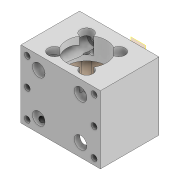
# Autodesk Inventor part: 30_Linear_Captive_Nema8_Guidemount
Saved by Autodesk Inventor 2022 (Build 260153000, 153)
## iProperties
Created: 2022-12-17
Part Number: 30_Linear_Captive_Nema8_Guidemount
Material: Generisch
Document SubType Name: Modeling
Designer: diederichbenedict
Density: 1 g/cm^3
Appearance: Vorgabe
Author: diederichbenedict
Autodesk Inventor part; units mm, degrees
ref_plane "YZ Plane" through (0, 0, 0) normal (1, 0, 0) x (0, 1, 0)
ref_plane "Arbeitsebene1" through (19.299985, 0, -3) normal (0, 0, 1) x (1, 0, 0)
ref_plane "Arbeitsebene2" through (22.999982, -10.5, 0) normal (0, 1, 0) x (-1, 0, 0)
ref_plane "Arbeitsebene3" through (-0.600008, 0, -10) normal (0, 1, 0) x (0, 0, 1)
sketch "Skizze1" plane through (22.999982, -10.5, 0) normal (0, 1, 0) x (-1, 0, 0)
  circle A0 centre (10.1, 12.1) radius 9.4488
  line L0 (0, 19.9) -> (0, 4.3)
  circle A1 centre (2.4, 4.4) radius 1
  circle A2 centre (2.4, 19.8) radius 1
  circle A3 centre (17.8, 19.8) radius 1
  circle A4 centre (17.8, 4.4) radius 1
  arc A5 (4.255177, -11.626563) -> (4.832799, -11.127251) centre (3.800005, -10.516241) ccw
  arc A6 (5.026176, -11.005497) -> (4.832799, -11.127251) centre (5.047965, -11.254545) ccw
  line L1 (5.026176, -11.005497) -> (5.371793, -10.975259)
  arc A7 (5.371793, -10.975259) -> (5.600004, -10.726211) centre (5.350004, -10.726211) ccw
  line L2 (5.600004, -10.726211) -> (5.600004, -10.273789)
  arc A8 (5.600004, -10.273789) -> (5.371793, -10.024741) centre (5.350004, -10.273789) ccw
  line L3 (5.371793, -10.024741) -> (5.005228, -9.992671)
  arc A9 (4.815463, -9.876832) -> (5.005228, -9.992671) centre (5.027016, -9.743622) ccw
  arc A10 (4.815463, -9.876832) -> (4.255177, -9.405918) centre (3.800005, -10.516241) ccw
  arc A11 (4.100005, -9.174601) -> (4.255177, -9.405918) centre (4.350005, -9.174601) ccw
  line L4 (4.100005, -9.174601) -> (4.100005, -8.500004)
  line L5 (4.100005, -8.500004) -> (4.600004, -8.000004)
  line L6 (4.600004, -8.000004) -> (15.599996, -8.000004)
  line L7 (15.599996, -8.000004) -> (16.099995, -8.500004)
  line L8 (16.099995, -8.500004) -> (16.099995, -9.174601)
  arc A12 (15.944823, -9.405918) -> (16.099995, -9.174601) centre (15.849995, -9.174601) ccw
  arc A13 (15.944823, -9.405918) -> (15.384537, -9.876832) centre (16.399995, -10.516241) ccw
  arc A14 (15.194772, -9.992671) -> (15.384537, -9.876832) centre (15.172984, -9.743622) ccw
  line L9 (15.194772, -9.992671) -> (14.828207, -10.024741)
  arc A15 (14.828207, -10.024741) -> (14.599996, -10.273789) centre (14.849996, -10.273789) ccw
  line L10 (14.599996, -10.273789) -> (14.599996, -10.726211)
  arc A16 (14.599996, -10.726211) -> (14.828207, -10.975259) centre (14.849996, -10.726211) ccw
  line L11 (14.828207, -10.975259) -> (15.173824, -11.005497)
  arc A17 (15.367201, -11.127251) -> (15.173824, -11.005497) centre (15.152035, -11.254545) ccw
  arc A18 (15.367201, -11.127251) -> (15.944823, -11.626563) centre (16.399995, -10.516241) ccw
  arc A19 (16.099995, -11.85788) -> (15.944823, -11.626563) centre (15.849995, -11.85788) ccw
  line L12 (16.099995, -11.85788) -> (16.099995, -13)
  line L13 (16.099995, -13) -> (22.99999, -13)
  line L14 (22.99999, -13) -> (23.599989, -12.4)
  line L15 (23.599989, -12.4) -> (23.599989, -9.000003)
  arc A20 (23.599989, -8.200004) -> (23.599989, -9.000003) centre (23.899989, -8.600004) ccw
  line L16 (23.599989, -8.200004) -> (23.599989, -3.600008)
  line L17 (23.599989, -3.600008) -> (22.999982, -3)
  line L18 (22.999982, -3) -> (16.500003, -3)
  line L19 (16.500003, -3) -> (16.099995, -3.400008)
  line L20 (16.099995, -3.400008) -> (4.100005, -3.400008)
  line L21 (4.100005, -3.400008) -> (3.699997, -3)
  line L22 (3.699997, -3) -> (-2.799982, -3)
  line L23 (-2.799982, -3) -> (-3.399989, -3.600008)
  line L24 (-3.399989, -3.600008) -> (-3.399989, -12.4)
  line L25 (-3.399989, -12.4) -> (-2.79999, -13)
  line L26 (-2.79999, -13) -> (4.100005, -13)
  line L27 (4.100005, -13) -> (4.100005, -11.85788)
  arc A21 (4.255177, -11.626563) -> (4.100005, -11.85788) centre (4.350005, -11.85788) ccw
  line L28 (-4.408908, -2.991081) -> (23.599989, -2.991081)
  line L29 (23.599989, -2.991081) -> (23.599989, 25.008919)
  line L30 (23.599989, 25.008919) -> (-4.408908, 25.008919)
  line L31 (-4.408908, 25.008919) -> (-4.408908, -2.991081)
  line L32 (-4.408908, 25.008919) -> (-9.408908, 25.008919)
  line L33 (-9.408908, 25.008919) -> (-9.408908, -2.991081)
  line L34 (-9.408908, -2.991081) -> (-4.408908, -2.991081)
  line L35 (-4.408908, -2.991081) -> (-4.408908, 25.008919)
  line L36 (23.599989, 25.008919) -> (28.599989, 25.008919)
  line L37 (28.599989, 25.008919) -> (28.599989, -2.991081)
  line L38 (28.599989, -2.991081) -> (23.599989, -2.991081)
  line L39 (23.599989, -2.991081) -> (23.599989, 25.008919)
  point P0 (-4.408908, -2.991081)
extrude "Extrusion1" add sketch "Skizze1" along normal up to surface (10.5 mm away) contours L31 L30 L29 L28 | L34 L33 L32 L31 | L29 L36 L37 L38
sketch "Skizze2" plane through (22.999982, -10.5, 0) normal (0, -1, 0) x (1, 0, 0)
  line L0 (0, 19.9) -> (0, 4.3)
  arc A0 (-2.3, 2) -> (0, 4.3) centre (-2.3, 4.3) ccw
  line L1 (-2.3, 2) -> (-17.9, 2)
  arc A1 (-20.2, 4.3) -> (-17.9, 2) centre (-17.9, 4.3) ccw
  line L2 (-20.2, 4.3) -> (-20.2, 19.9)
  arc A2 (-17.9, 22.2) -> (-20.2, 19.9) centre (-17.9, 19.9) ccw
  line L3 (-17.9, 22.2) -> (-2.3, 22.2)
  arc A3 (0, 19.9) -> (-2.3, 22.2) centre (-2.3, 19.9) ccw
  circle A4 centre (-10.1, 12.1) radius 8
  circle A5 centre (-2.4, 4.4) radius 1
  circle A6 centre (-17.8, 4.4) radius 1
  circle A7 centre (-17.8, 19.8) radius 1
  circle A8 centre (-2.4, 19.8) radius 1
  line L4 (0.2, 4.3) -> (0.2, 19.9)
  arc A9 (0.2, 19.9) -> (-2.3, 22.4) centre (-2.3, 19.9) ccw
  line L5 (-2.3, 22.4) -> (-17.9, 22.4)
  arc A10 (-17.9, 22.4) -> (-20.4, 19.9) centre (-17.9, 19.9) ccw
  line L6 (-20.4, 19.9) -> (-20.4, 4.3)
  arc A11 (-20.4, 4.3) -> (-17.9, 1.8) centre (-17.9, 4.3) ccw
  line L7 (-17.9, 1.8) -> (-2.3, 1.8)
  arc A12 (-2.3, 1.8) -> (0.2, 4.3) centre (-2.3, 4.3) ccw
  circle A13 centre (-10.1, 12.1) radius 1.75
  circle A14 centre (-17.8, 4.4) radius 1
  circle A15 centre (-17.8, 19.8) radius 1
  circle A16 centre (-2.4, 19.8) radius 1
  circle A17 centre (-2.4, 4.4) radius 1
  circle A18 centre (-10.1, 12.1) radius 9.4488
  circle A19 centre (-10.1, 12.1) radius 9.4488
  circle A20 centre (-2.4, 4.4) radius 1
  circle A21 centre (-2.4, 19.8) radius 1
  circle A22 centre (-17.8, 19.8) radius 1
  circle A23 centre (-17.8, 4.4) radius 1
  line L8 (-28.599989, 25.008919) -> (9.408908, 25.008919)
  line L9 (-28.599989, -2.991081) -> (-28.599989, 25.008919)
  line L10 (9.408908, -2.991081) -> (-28.599989, -2.991081)
  line L11 (9.408908, 25.008919) -> (9.408908, -2.991081)
  circle A24 centre (-17.8, 4.4) radius 1
  circle A25 centre (-17.8, 19.8) radius 1
  circle A26 centre (-2.4, 19.8) radius 1
  circle A27 centre (-2.4, 4.4) radius 1
  circle A28 centre (-10.1, 12.1) radius 9.4488
  point P0 (-22.999982, 0)
  dimension "d3" = 0.2
  constraints: 8 end point, 8 point on circle, 4 centre point, 7 other
  measures "d3" distance between parallel lines of L0 L4
ref_plane "Arbeitsebene4" through (-0.600008, -32.4, -10) normal (0, -1, 0) x (1, 0, 0)
extrude "Extrusion2" add sketch "Skizze2" along normal up to surface (21.9 mm away) contours L8 L11 L10 L9
sketch "Skizze3" plane through (0.899971, 0, -0.400008) normal (0, 1, 0) x (1, 0, 0)
  circle A0 centre (12.000011, -12.500008) radius 9.4488
  circle A1 centre (19.700011, -4.800008) radius 1
  circle A2 centre (19.700011, -20.200008) radius 1
  circle A3 centre (4.300011, -20.200008) radius 1
  circle A4 centre (4.300011, -4.800008) radius 1
  point P0 (-0.899971, -0.400008)
hole "Bohrung1" at (20.599982, 0, 4.4) at (20.599982, 0, 19.8) at (5.199982, 0, 19.8) at (5.199982, 0, 4.4) direction (0, -1, 0) diameter 2.5 end through all counterbore diameter 6 counterbore depth 8
sketch "Skizze4" plane through (0.899971, 0, 25.008919) normal (0, 0, 1) x (1, 0, 0)
  circle A0 centre (22.000011, -6.2) radius 1.25
  circle A1 centre (22.000011, -26.2) radius 1.25
  circle A2 centre (2.000011, -26.2) radius 1.25
  circle A3 centre (2.000011, -6.2) radius 1.25
  point P0 (-0.899971, 0)
hole "Bohrung2" at (2.899982, -26.2, 25.008919) at (2.899982, -6.2, 25.008919) at (22.899982, -26.2, 25.008919) at (22.899982, -6.2, 25.008919) direction (0, 0, -1) diameter 2.8 end through all counterbore diameter 6 counterbore depth 26
sketch "Skizze7" plane through (-5.600008, 0, 25.008919) normal (0, 0, 1) x (1, 0, 0)
  circle A0 centre (28.499989, -26.2) radius 3
  circle A1 centre (8.499989, -26.2) radius 3
  circle A2 centre (8.499989, -6.2) radius 3
  circle A3 centre (28.499989, -6.2) radius 3
  line L0 (38.008897, 0) -> (0, 0)
  line L1 (0, 0) -> (0, -32.4)
  line L2 (0, -32.4) -> (38.008897, -32.4)
  line L3 (38.008897, -32.4) -> (38.008897, 0)
  line L4 (35.008897, -29.4) -> (3, -29.4) construction
  line L5 (3, -29.4) -> (3, -3) construction
  line L6 (3, -3) -> (35.008897, -3) construction
  line L7 (35.008897, -3) -> (35.008897, -29.4) construction
  circle A4 centre (16.2, -16.2) radius 13.2
  point P0 (5.600008, 0)
  point P1 (35.008897, -16.2)
  point P2 (3, -16.2)
  dimension "d26" = 3
  dimension "d42" = 32.0089
  dimension "d43" = 26.4
  dimension "d44" = 32.4
  dimension "d45" = 3
  constraints: 8 end point, 3 tangent, 2 midpoint, 1 centre point, 3 other
  measures "d26" distance between parallel lines of L2 L4
  measures "d42" distance of L6.end L5.end
  measures "d43" distance of L4.start L6.end
  measures "d44" distance between parallel lines of L2 L0
  measures "d45" distance from line of L5.end L1
hole "Bohrung3" at (29.408889, -29.4, 25.008919) at (-2.600008, -29.4, 25.008919) at (-2.600008, -3, 25.008919) at (29.408889, -3, 25.008919) at (29.408889, -16.2, 25.008919) at (-2.600008, -16.2, 25.008919) direction (0, 0, -1) diameter 2.8 end through all
sketch "Skizze8" plane through (-5.600008, 0, -2.991081) normal (-1, 0, 0) x (0, 0, 1)
  line L0 (28, 0) -> (0, 0) projected
  line L1 (0, -32.4) -> (0, 0) projected
  line L2 (0, -32.4) -> (28, -32.4) projected
  line L3 (28, 0) -> (28, -32.4) projected
  line L4 (25, -29.4) -> (3, -29.4) construction
  line L5 (3, -29.4) -> (3, -3) construction
  line L6 (3, -3) -> (25, -3) construction
  line L7 (25, -3) -> (25, -29.4) construction
  circle A0 centre (16.2, -16.2) radius 13.2
  point P0 (2.991081, 0)
  point P1 (25, -16.2)
  point P2 (3, -16.2)
  dimension "d34" = 3
  constraints: 8 end point, 2 horizontal, 2 midpoint, 1 horizontal alignment, 1 vertical, 5 other
  measures "d34" distance between parallel lines of L2 L4
hole "Bohrung4" at (-5.600008, -16.2, 22.008919) at (-5.600008, -16.2, 0.008919) at (-5.600008, -29.4, 22.008919) at (-5.600008, -29.4, 0.008919) at (-5.600008, -3, 0.008919) at (-5.600008, -3, 22.008919) direction (1, 0, 0) diameter 2.8 depth 8 tip angle 118
